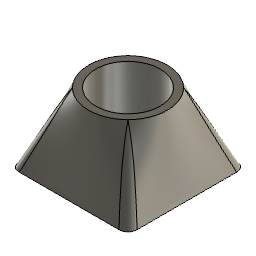
APC5000_Battery_Stand_v1 (Autodesk Fusion 360 design; units mm, degrees)
part number: 2026-02-11-11-32-26-972
Autodesk Fusion 360 part; units mm, degrees
sketch "Sketch1" plane through (0, 0, 0) normal (0, 0, 1) x (1, 0, 0)
  line L0 (-30, 30) -> (30, 30)
  line L1 (30, 30) -> (30, -30)
  line L2 (30, -30) -> (-30, -30)
  line L3 (-30, -30) -> (-30, 30)
  line L4 (-30, 30) -> (30, -30) construction
  line L5 (30, 30) -> (-30, -30) construction
  dimension "d6" = 60
  dimension "d7" = 60
  constraint horizontal L0
  constraint perpendicular L0 L1
  constraint parallel L0 L2
  constraint parallel L1 L3
  constraint coincident L4 origin
  constraint coincident L5 origin
  measures "d6" distance of L1.end L2.end
  measures "d7" distance of L0.end L1.end
ref_plane "WorkPlane1" through (0, 0, 35) normal (0, 0, 1) x (1, 0, 0)
sketch "Sketch2" plane through (0, 0, 35) normal (0, 0, 1) x (1, 0, 0)
  circle A0 centre (0, 0) radius 20
  dimension "d10" = 40
  constraint coincident A0.centre origin
  measures "d10" diameter of A0
loft "Loft1" add profiles "Sketch1", "Sketch2" section 1 section 2
sketch "Sketch3" plane through (0, 0, 35) normal (0, 0, 1) x (-1, 0, 0)
  arc A0 (14.1421, 14.1421) -> (-14.1421, 14.1421) centre (0, 0) ccw
  arc A1 (-14.1421, 14.1421) -> (-14.1421, -14.1421) centre (0, 0) ccw
  arc A2 (-14.1421, -14.1421) -> (14.1421, -14.1421) centre (0, 0) ccw
  arc A3 (14.1421, -14.1421) -> (14.1421, 14.1421) centre (0, 0) ccw
  circle A4 centre (0, 0) radius 16.375
  dimension "d11" = 32.75
  constraint concentric A0 A4
  measures "d11" diameter of A4
extrude "Extrude1" cut sketch "Sketch3" against normal blind 25 contours A4
fillet "Fillet1" radius 5 4 edges at (-22.0711, 22.0711, 17.5) (22.0711, 22.0711, 17.5) (22.0711, -22.0711, 17.5) (-22.0711, -22.0711, 17.5)
equation "hole_diameter = 32.75 mm" comment "was 32.50"
equation "hole_depth = 25 mm"
equation "flange_height = 10 mm"
equation "square_base = 60 mm"
equation "circular_top = 40 mm"
equation "d6 = square_base"
equation "d7 = square_base"
equation "total_height = flange_height + hole_depth"
equation "d9 = total_height"
equation "d10 = circular_top"
equation "d11 = hole_diameter"
equation "d12 = -hole_depth"
equation "filet_mm = 5 mm"
equation "d16 = filet_mm"
